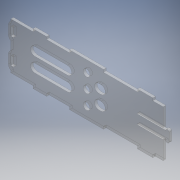
# Autodesk Inventor part: Bottom_plate2
Saved by Autodesk Inventor 2016 (Build 200138000, 138)
## iProperties
Created: 2015-07-16
Part Number: Bottom_plate2
Material: Polycarbonate, Clear
Document SubType Name: Modeling
Designer: Openlab
Density: 1.2 g/cm^3
Appearance: Polycarbonate - Clear
Author: Openlab
Autodesk Inventor part; units mm, degrees
ref_plane "YZ Plane" through (0, 0, 0) normal (1, 0, 0) x (0, 1, 0)
ref_plane "XZ Plane" through (0, 0, 0) normal (0, 1, 0) x (-1, 0, 0)
ref_plane "XY Plane" through (0, 0, 0) normal (0, 0, 1) x (1, 0, 0)
sketch "Sketch1" plane through (0, 0, 0) normal (0, 1, 0) x (-1, 0, 0)
  line L0 (37.25, -2.25) -> (24.75, -2.25) construction
  line L1 (24.75, -2.25) -> (24.75, -14.75) construction
  line L2 (24.75, -14.75) -> (37.25, -14.75) construction
  line L3 (37.25, -14.75) -> (37.25, -2.25) construction
  line L4 (56.9183, -8.5) -> (8.3915, -8.5) construction
  line L5 (0, -17) -> (105, -17) construction
  line L6 (0, 0) -> (0, -51) construction
  line L7 (0, -34) -> (105, -34) construction
  line L8 (105, -51) -> (105, 0) construction
  line L9 (31, 55.8243) -> (31, -51) construction
  line L10 (56.8064, -25.5) -> (17, -25.5) construction
  line L11 (24.75, -19.25) -> (24.75, -31.75) construction
  line L12 (37.25, -19.25) -> (24.75, -19.25) construction
  line L13 (37.25, -31.75) -> (37.25, -19.25) construction
  line L14 (24.75, -31.75) -> (37.25, -31.75) construction
  line L15 (24.75, -36.25) -> (24.75, -48.75) construction
  line L16 (37.25, -36.25) -> (24.75, -36.25) construction
  line L17 (37.25, -48.75) -> (37.25, -36.25) construction
  line L18 (24.75, -48.75) -> (37.25, -48.75) construction
  line L19 (56.3008, -42.5) -> (16.5498, -42.5) construction
  arc A0 (53.45, -12) -> (53.45, -22) centre (53.45, -17) ccw
  arc A1 (92, -22) -> (92, -12) centre (92, -17) ccw
  arc A2 (53.45, -29) -> (53.45, -39) centre (53.45, -34) ccw
  arc A3 (92, -39) -> (92, -29) centre (92, -34) ccw
  line L20 (53.45, -12) -> (92, -12)
  line L21 (53.45, -22) -> (92, -22)
  line L22 (53.45, -29) -> (92, -29)
  line L23 (53.45, -39) -> (92, -39)
  arc A4 (16.65, -39) -> (16.65, -29) centre (16.65, -34) ccw
  line L24 (103.5, -49.5) -> (103.5, -1.5) construction
  line L25 (1.5, -1.5) -> (1.5, -49.5) construction
  arc A5 (14, -29) -> (14, -39) centre (14, -34) ccw
  arc A6 (14, -12) -> (14, -22) centre (14, -17) ccw
  line L26 (16.65, -39) -> (14, -39)
  line L27 (14, -29) -> (16.65, -29)
  line L28 (14, -22) -> (16.65, -22)
  line L29 (16.65, -12) -> (14, -12)
  arc A7 (16.65, -22) -> (16.65, -12) centre (16.65, -17) ccw
  arc A8 (96.5, -51) -> (93, -47.5) centre (93, -51) ccw construction
  arc A9 (53.45, -47.5) -> (49.95, -51) centre (53.45, -51) ccw construction
  arc A10 (97.7697, -49.5) -> (93, -46) centre (93, -51) ccw construction
  line L30 (93, -46) -> (53.45, -46) construction
  line L31 (96.5, -51) -> (105, -51) construction
  line L32 (93, -47.5) -> (53.45, -47.5) construction
  line L33 (105, -49.5) -> (97.7697, -49.5) construction
  arc A11 (53.45, -46) -> (48.6803, -49.5) centre (53.45, -51) ccw construction
  arc A12 (48.6803, -1.5) -> (53.45, -5) centre (53.45, 0) ccw construction
  arc A13 (49.95, 0) -> (53.45, -3.5) centre (53.45, 0) ccw construction
  line L34 (93, -3.5) -> (53.45, -3.5) construction
  line L35 (93, -5) -> (53.45, -5) construction
  line L36 (97.7697, -1.5) -> (105, -1.5) construction
  line L37 (105, 0) -> (96.5, 0) construction
  arc A14 (93, -3.5) -> (96.5, 0) centre (93, 0) ccw construction
  arc A15 (93, -5) -> (97.7697, -1.5) centre (93, 0) ccw construction
  arc A16 (16.65, -51) -> (13.15, -47.5) centre (13.15, -51) ccw construction
  arc A17 (12, -47.5) -> (8.5, -51) centre (12, -51) ccw construction
  line L38 (13.15, -46) -> (12, -46) construction
  line L39 (13.15, -47.5) -> (12, -47.5) construction
  arc A18 (12, -46) -> (7.2303, -49.5) centre (12, -51) ccw construction
  arc A19 (17.9197, -49.5) -> (13.15, -46) centre (13.15, -51) ccw construction
  line L40 (48.6803, -49.5) -> (17.9197, -49.5) construction
  line L41 (7.2303, -49.5) -> (0, -49.5) construction
  line L42 (0, -51) -> (8.5, -51) construction
  line L43 (16.65, -51) -> (49.95, -51) construction
  line L44 (13.15, -5) -> (12, -5) construction
  line L45 (13.15, -3.5) -> (12, -3.5) construction
  arc A20 (8.5, 0) -> (12, -3.5) centre (12, 0) ccw construction
  arc A21 (13.15, -3.5) -> (16.65, 0) centre (13.15, 0) ccw construction
  arc A22 (7.2303, -1.5) -> (12, -5) centre (12, 0) ccw construction
  arc A23 (13.15, -5) -> (17.9197, -1.5) centre (13.15, 0) ccw construction
  line L46 (49.95, 0) -> (16.65, 0) construction
  line L47 (8.5, 0) -> (0, 0) construction
  line L48 (0, -1.5) -> (7.2303, -1.5) construction
  line L49 (17.9197, -1.5) -> (48.6803, -1.5) construction
  arc A24 (38.75, -4.25) -> (35.25, -0.75) centre (35.25, -4.25) ccw construction
  arc A25 (26.75, -0.75) -> (23.25, -4.25) centre (26.75, -4.25) ccw construction
  arc A26 (35.25, -50.25) -> (38.75, -46.75) centre (35.25, -46.75) ccw construction
  arc A27 (23.25, -46.75) -> (26.75, -50.25) centre (26.75, -46.75) ccw construction
  line L50 (38.75, -4.25) -> (38.75, -46.75) construction
  line L51 (35.25, -0.75) -> (26.75, -0.75) construction
  line L52 (23.25, -4.25) -> (23.25, -46.75) construction
  line L53 (26.75, -50.25) -> (35.25, -50.25) construction
  line L54 (51, 5) -> (51, 2)
  line L55 (78, 5) -> (78, 2)
  line L56 (94, 5) -> (94, 2)
  line L57 (11, 5) -> (11, 2)
  line L58 (-29, 2) -> (-29, 5)
  line L59 (51, -56) -> (51, -53)
  line L60 (11, -56) -> (11, -53)
  line L61 (-29, -56) -> (-29, -53)
  line L62 (78, -56) -> (78, -53)
  line L63 (94, -56) -> (94, -53)
  line L64 (-47, 5) -> (-47, 2)
  line L65 (-47, -53) -> (-47, -56)
  line L66 (11, 2) -> (-29, 2)
  line L67 (120, 2) -> (94, 2)
  line L68 (78, 2) -> (51, 2)
  line L69 (51, -53) -> (78, -53)
  line L70 (94, -53) -> (120, -53)
  line L71 (-29, -53) -> (11, -53)
  line L72 (-47, 2) -> (-59, 2)
  line L73 (-59, -53) -> (-47, -53)
  circle A28 centre (31, -8.5) radius 4
  circle A29 centre (31, -25.5) radius 4
  circle A30 centre (31, -42.5) radius 4
  line L74 (51, 5) -> (11, 5)
  line L75 (-29, 5) -> (-47, 5)
  line L76 (-47, -56) -> (-29, -56)
  line L77 (11, -56) -> (51, -56)
  line L78 (78, -56) -> (94, -56)
  line L79 (-59, 2) -> (-59, -19.5)
  line L80 (-59, -31.5) -> (-59, -53)
  line L81 (120, -5.5) -> (117, -5.5)
  line L82 (117, -5.5) -> (117, -15.5)
  line L83 (117, -15.5) -> (120, -15.5)
  line L84 (120, -15.5) -> (120, -5.5)
  line L85 (120, -35.5) -> (117, -35.5)
  line L86 (117, -35.5) -> (117, -45.5)
  line L87 (117, -45.5) -> (120, -45.5)
  line L88 (120, -45.5) -> (120, -35.5)
  line L89 (-59, -19.5) -> (-29, -19.5)
  arc A31 (-29, -20.5) -> (-29, -19.5) centre (-29, -20) ccw
  line L90 (-29, -20.5) -> (-62, -20.5)
  line L91 (-62, -30.5) -> (-29, -30.5)
  arc A32 (-29, -31.5) -> (-29, -30.5) centre (-29, -31) ccw
  line L92 (-59, -31.5) -> (-29, -31.5)
  arc A33 (-62, -20.5) -> (-66, -20.5) centre (-64, -20.5) ccw
  arc A34 (-66, -30.5) -> (-62, -30.5) centre (-64, -30.5) ccw
  line L93 (-66, -30.5) -> (-66, -20.5)
  arc A35 (120, -50.6962) -> (123, -45.5) centre (117, -45.5) ccw
  arc A36 (123, -5.5) -> (120, -0.3038) centre (117, -5.5) ccw
  line L94 (120, -0.3038) -> (120, 2)
  line L95 (120, -50.6962) -> (120, -53)
  arc A37 (123, -35.5) -> (120, -30.3038) centre (117, -35.5) ccw
  arc A38 (120, -20.6962) -> (123, -15.5) centre (117, -15.5) ccw
  line L96 (120, -20.6962) -> (120, -30.3038)
  line L97 (123, -45.5) -> (123, -35.5)
  line L98 (123, -15.5) -> (123, -5.5)
  line L99 (94, 5) -> (78, 5)
  dimension "d0" = 12.5
  dimension "d1" = 12.5
  dimension "d2" = 17
  dimension "d3" = 31
  dimension "d4" = 105
  dimension "d5" = 17
  dimension "d6" = 17
  dimension "d7" = 10
  dimension "d8" = 1.5
  dimension "d9" = 1.5
  dimension "d10" = 5
  dimension "d11" = 1.5
  dimension "d12" = 1.5
  dimension "d13" = 1.5
  dimension "d14" = 17
  dimension "d15" = 17
  dimension "d16" = 12
  dimension "d17" = 13
  dimension "d18" = 11.6
  dimension "d19" = 12
  dimension "d20" = 2
  dimension "d21" = 2
  dimension "d22" = 7
  dimension "d23" = 2
  dimension "d24" = 2
  dimension "d25" = 40
  dimension "d26" = 40
  dimension "d27" = 18
  dimension "d30" = 2
  dimension "d31" = 14
  dimension "d32" = 8.1
  dimension "d33" = 22.45
  dimension "d38" = 55
  dimension "d39" = 8
  dimension "d46" = 3
  dimension "d52" = 12
  dimension "d53" = 10
  dimension "d54" = 3
  dimension "d56" = 20
  dimension "d57" = 30
  dimension "d58" = 1
  dimension "d59" = 10
  dimension "d60" = 4
  dimension "d62" = 3
  dimension "d64" = 3
  dimension "d67" = 27
  dimension "d68" = 16
  dimension "d71" = 26
  constraints: 200 end point, 72 point on circle, 54 perpendicular, 45 tangent, 39 centre point, 32 point on line, 31 collinear, 31 parallel, 28 equal radius, 21 horizontal, 18 coincident, 14 vertical alignment, 10 equal length, 9 horizontal alignment, 2 vertical, 13 other
  measures "d0" distance of L2.end L1.end
  measures "d1" distance of L0.end L1.end
  measures "d2" distance between parallel lines of L10 L4
  measures "d3" distance between parallel lines of L6 L9
  measures "d4" distance between parallel lines of L6 L8
  measures "d5" distance between parallel lines of L19 L10
  measures "d6" distance between parallel lines of L5 L7
  measures "d7" diameter of A0
  measures "d8" distance between parallel lines of L6 L25
  measures "d9" distance between parallel lines of L8 L24
  measures "d10" radius of A4
  measures "d11" radial gap between concentric circles of A8 A10
  measures "d12" distance between parallel lines of L37 L36
  measures "d13" distance between parallel lines of L41 L42
  measures "d14" distance between parallel lines of L7 L42
  measures "d15" distance between parallel lines of L47 L5
  measures "d16" distance from line of A8.centre L8
  measures "d17" distance from line of L8 A3.centre
  measures "d18" distance from line of A19.centre L15
  measures "d19" distance from line of L6 A22.centre
  measures "d20" distance from line of L1 A25.centre
  measures "d21" distance from line of A25.centre L0
  measures "d22" diameter of A25
  measures "d23" distance from line of L17 A26.centre
  measures "d24" distance from line of L18 A26.centre
  measures "d25" distance between parallel lines of L57 L54
  measures "d26" distance between parallel lines of L58 L57
  measures "d27" distance between parallel lines of L64 L58
  measures "d30" distance between parallel lines of L67 L37
  measures "d31" distance from line of L6 A5.centre
  measures "d32" distance from line of L15 A4.centre
  measures "d33" distance from line of L9 A9.centre
  measures "d38" distance between parallel lines of L70 L67
  measures "d39" diameter of A28
  measures "d46" distance of L65.start L65.end
  measures "d52" distance between parallel lines of L79 L64
  measures "d53" distance of L81.end L82.end
  measures "d54" distance of L81.start L81.end
  measures "d56" distance between parallel lines of L85 L83
  measures "d57" distance from line of L79 A31.centre
  measures "d58" diameter of A31
  measures "d59" distance between parallel lines of L91 L90
  measures "d60" diameter of A34
  measures "d62" distance from line of L90.end L79
  measures "d64" distance between parallel lines of L98 L84
  measures "d67" distance between parallel lines of L54 L55
  measures "d68" distance between parallel lines of L55 L56
  measures "d71" distance between parallel lines of L56 L94
extrude "Extrusion1" add sketch "Sketch1" along normal blind 3
body "Solid1"
